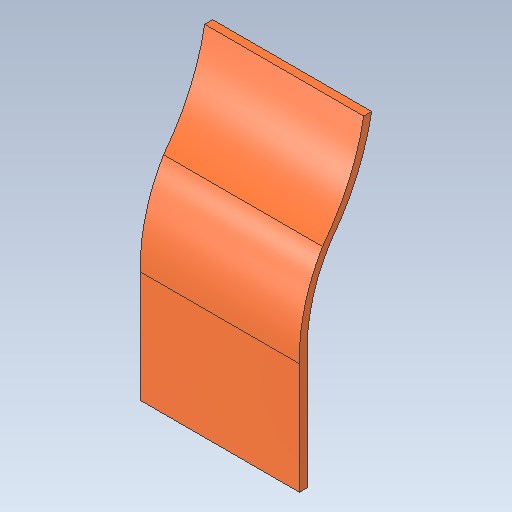
# Autodesk Inventor part: ribbonCable
Saved by Autodesk Inventor 2020 (Build 240168000, 168)
## iProperties
Created: 2018-12-01
Part Number: ribbonCable
Material: Generic
Document SubType Name: Modeling
Designer: Ralf
Density: 1 g/cm^3
Appearance: Default
Author: Ralf
Autodesk Inventor part; units mm, degrees
ref_plane "YZ Plane" through (0, 0, 0) normal (1, 0, 0) x (0, 1, 0)
ref_plane "XZ Plane" through (0, 0, 0) normal (0, 1, 0) x (-1, 0, 0)
ref_plane "XY Plane" through (0, 0, 0) normal (0, 0, 1) x (1, 0, 0)
sketch "Sketch1" plane through (0, 0, 0) normal (1, 0, 0) x (0, 1, 0)
  line L0 (0, 0) -> (3.5, 0)
  arc A0 (6.3262, -0.7277) -> (3.5, 0) centre (3.7831, -4.7528) ccw
  arc A1 (6.3262, -0.7277) -> (9.2314, -2.0228) centre (10.456, 4.6303) ccw
  line L1 (0, 0) -> (0, 0.25)
  line L2 (0, 0.25) -> (3.5, 0.25)
  line L3 (6.3262, -0.7277) -> (6.3262, -0.4777)
  line L4 (9.2314, -2.0228) -> (9.2314, -1.7728)
  arc A2 (6.3262, -0.4777) -> (3.5, 0.25) centre (3.658, -4.9886) ccw
  arc A3 (6.3262, -0.4777) -> (9.2314, -1.7728) centre (10.4213, 4.8026) ccw
  dimension "d0" = 3.5
  dimension "d1" = 0.25
  dimension "d2" = 3.5
  dimension "d3" = 0.25
  dimension "d4" = 0.25
  constraints: 10 end point, 8 point on circle, 4 centre point, 3 vertical, 2 horizontal
  measures "d0" distance of L0.start L0.end
  measures "d1" distance of L0.start L1.end
  measures "d2" distance of L1.end L2.end
  measures "d3" distance of L3.start L3.end
  measures "d4" distance of L4.start L4.end
extrude "Extrusion1" add sketch "Sketch1" along normal blind 5
body "Solid1"
